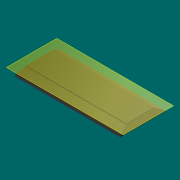
# Autodesk Inventor part: edgeCoating
Saved by Autodesk Inventor 2016 (Build 200138000, 138)
## iProperties
Created: 2016-02-15
Part Number: edgeCoating
Material: Rubber
Document SubType Name: Modeling
Designer: sawai
Density: 0.93 g/cm^3
Appearance: Rubber - Black
Author: sawai
Autodesk Inventor part; units mm, degrees
ref_plane "YZ Plane" through (0, 0, 0) normal (1, 0, 0) x (0, 1, 0)
ref_plane "XZ Plane" through (0, 0, 0) normal (0, 1, 0) x (-1, 0, 0)
sketch "Sketch1" plane through (0, 0, 0) normal (0, 0, 1) x (1, 0, 0)
  line L0 (-5.7, 5.7) -> (5.7, 5.7) projected
  line L1 (-5.7, -5.7) -> (-5.7, 5.7) projected
  line L2 (5.7, -5.7) -> (-5.7, -5.7) projected
  line L3 (5.7, 5.7) -> (5.7, -5.7) projected
  point P0 (0, 0)
ref_plane "Work Plane1" through (0, 0, 1.45) normal (0, 0, 1) x (1, 0, 0)
sketch "Sketch2" plane through (0, 0, 1.45) normal (0, 0, 1) x (1, 0, 0)
  line L0 (12.5, 3.5) -> (-12.5, 3.5) projected
  line L1 (-12.5, 3.5) -> (-12.5, -3.5) projected
  line L2 (-12.5, -3.5) -> (12.5, -3.5) projected
  line L3 (12.5, -3.5) -> (12.5, 3.5) projected
  point P0 (0, 0)
loft "Loft1" add profiles "Sketch2", "Sketch1"
sketch "Sketch3" plane through (-12.5, 3.5, 1.45) normal (0, 0, 1) x (1, 0, 0)
  line L0 (0, 0) -> (0, -7) projected
  line L1 (25, 0) -> (0, 0) projected
  line L2 (25, -7) -> (25, 0) projected
  line L3 (0, -7) -> (25, -7) projected
  point P0 (12.5, -3.5)
extrude "Extrusion1" cut sketch "Sketch3" against normal through all
body "Solid1"
